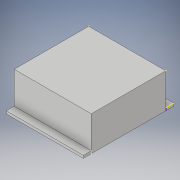
# Autodesk Inventor part: robotics battery box
Saved by Autodesk Inventor 2018 (Build 220112000, 112)
## iProperties
Created: 2018-01-20
Part Number: robotics battery box
Material: Generic
Document SubType Name: Modeling
Designer: kalra.rohan
Density: 1 g/cm^3
Appearance: Default
Author: kalra.rohan
Autodesk Inventor part; units mm, degrees
ref_plane "YZ Plane" through (0, 0, 0) normal (1, 0, 0) x (0, 1, 0)
ref_plane "XZ Plane" through (0, 0, 0) normal (0, 1, 0) x (-1, 0, 0)
ref_plane "XY Plane" through (0, 0, 0) normal (0, 0, 1) x (1, 0, 0)
sketch "Sketch1" plane through (0, 0, 0) normal (0, 0, 1) x (1, 0, 0)
  line L0 (0, 0) -> (184.15, 0)
  line L1 (184.15, 0) -> (184.15, -107.95)
  line L2 (184.15, -107.95) -> (0, -107.95)
  line L3 (0, -107.95) -> (0, 0)
  dimension "d0" = 107.95
  dimension "d1" = 184.15
  constraints: 8 end point, 2 parallel, 1 horizontal, 1 perpendicular
  measures "d0" distance between parallel lines of L2 L0
  measures "d1" distance between parallel lines of L1 L3
extrude "Extrusion1" add sketch "Sketch1" along normal blind 177.8
sketch "Sketch2" plane through (0, 0, 177.8) normal (0, 0, 1) x (1, 0, 0)
  line L0 (0, 0) -> (0, -107.95) projected
  line L1 (184.15, -107.95) -> (184.15, 0) projected
  line L2 (0, -76.2) -> (184.15, -76.2)
  line L3 (184.15, -76.2) -> (184.15, -82.55)
  line L4 (184.15, -82.55) -> (0, -82.55)
  line L5 (0, -82.55) -> (0, -76.2)
  line L6 (0, -107.95) -> (184.15, -107.95) projected
  dimension "d4" = 6.35
  dimension "d5" = 25.4
  constraints: 8 end point, 2 parallel, 2 point on line, 1 horizontal, 1 perpendicular
  measures "d4" distance between parallel lines of L4 L2
  measures "d5" distance between parallel lines of L6 L4
extrude "Extrusion2" add sketch "Sketch2" along normal blind 19.05 contours L2 L1 L4 L0
sketch "Sketch3" plane through (0, 0, 0) normal (0, 0, -1) x (-1, 0, 0)
  line L0 (0, -107.95) -> (0, 0) projected
  line L1 (-184.2181, -76.2) -> (0, -76.2)
  line L2 (0, -76.2) -> (0, -82.55)
  line L3 (0, -82.55) -> (-184.2181, -82.55)
  line L4 (-184.2181, -82.55) -> (-184.2181, -76.2)
  line L5 (-184.15, -107.95) -> (0, -107.95) projected
  line L6 (0, 0) -> (-184.15, 0) projected
  dimension "d8" = 25.4
  dimension "d9" = 76.2
  constraints: 8 end point, 2 parallel, 1 horizontal, 1 perpendicular, 1 point on line
  measures "d8" distance between parallel lines of L5 L3
  measures "d9" distance between parallel lines of L1 L6
extrude "Extrusion3" add sketch "Sketch3" along normal blind 19.05
sketch "Sketch4" plane through (184.15, 0, 177.8) normal (1, 0, 0) x (0, 0, -1)
  line L0 (177.8, -76.2) -> (177.8, -82.55)
  line L1 (177.8, -76.2) -> (196.85, -76.2) projected
  point P0 (177.8, 0)
  point P1 (0, -82.55)
  point P2 (0, -76.2)
  constraints: 2 end point
sketch "Sketch5" plane through (184.15, 0, 177.8) normal (1, 0, 0) x (0, 0, -1)
  point P0 (177.8, 0)
sketch "Sketch6" plane through (0, 0, 0) normal (0, 0, -1) x (-1, 0, 0)
  line L0 (-181.61, -2.54) -> (-2.54, -2.54)
  line L1 (-2.54, -2.54) -> (-2.54, -76.2)
  line L2 (-2.54, -76.2) -> (-181.61, -76.2)
  line L3 (-181.61, -76.2) -> (-181.61, -2.54)
  line L4 (0, 0) -> (-184.15, 0) projected
  line L5 (0, -76.2) -> (0, 0) projected
  line L6 (-184.15, 0) -> (-184.15, -76.2) projected
  line L7 (0, -76.2) -> (-184.2181, -76.2) projected
  dimension "d12" = 2.54
  dimension "d13" = 2.54
  dimension "d14" = 2.54
  dimension "d15" = 0
  constraints: 8 end point, 2 parallel, 1 horizontal, 1 perpendicular
  measures "d12" distance between parallel lines of L4 L0
  measures "d13" distance between parallel lines of L5 L1
  measures "d14" distance between parallel lines of L6 L3
  measures "d15" distance between parallel lines of L7 L2
extrude "Extrusion4" cut sketch "Sketch6" against normal blind 175.26 contours L0 L1 L2 L3
sketch "Sketch7" plane through (0, 0, 0) normal (0, 0, -1) x (-1, 0, 0)
  point P0 (0, 0)
sketch "Sketch8" plane through (0, 0, 0) normal (0, 0, -1) x (-1, 0, 0)
  line L0 (0, -82.55) -> (-184.15, -82.55) projected
  line L1 (-184.15, -82.55) -> (-184.15, -107.95) projected
  line L2 (-184.15, -107.95) -> (0, -107.95) projected
  line L3 (0, -107.95) -> (0, -82.55) projected
  point P0 (0, 0)
extrude "Extrusion5" cut sketch "Sketch8" against normal blind 177.8
body "Solid1"
